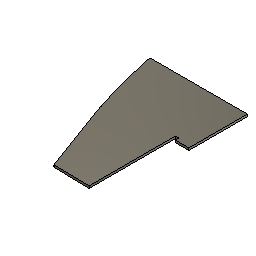
oceaan-25-floor_3 v6 (Autodesk Fusion 360 design; units mm, degrees)
Autodesk Fusion 360 part; units mm, degrees
note: some values were not read from the file. Set by a fixed rule: which sketch regions a step uses.
sketch "Sketch1" plane through (0, 0, 0) normal (0, 1, 0) x (1, 0, 0)
  line L0 (107.2779, 788.7865) -> (-437.7221, 788.7865)
  line L1 (12.2779, 481.7865) -> (31.2779, 481.7858)
  line L2 (31.2779, 481.7858) -> (31.1088, 461.7865)
  line L3 (31.1088, 461.7865) -> (107.2779, 461.7865)
  line L4 (12.2779, 481.7865) -> (12.2779, -0.2135)
  line L5 (-186.7221, 3.7865) -> (-186.7221, 419.7865)
  line L6 (-340.9767, 419.6292) -> (-188.1918, 3.7865)
  arc A0 (-437.7221, 788.7865) -> (-340.9767, 419.6292) centre (3793.4257, 1700.3924) ccw
  line L7 (12.2779, 788.7865) -> (107.2779, 788.7865)
  line L8 (12.2779, 788.7865) -> (107.2779, 788.7865)
  line L9 (107.2779, 788.7865) -> (107.2779, 481.7857)
  line L10 (107.2779, 481.7857) -> (107.2779, 461.7865)
  line L11 (12.2779, -0.2135) -> (-186.7221, 3.7865)
  line L12 (-186.7221, 3.7865) -> (-188.1918, 3.7865)
  dimension "d1" = 789
  dimension "d4" = 307
  dimension "d6" = 95
  dimension "d7" = 545
  dimension "d11" = 19
  dimension "d12" = 20
  dimension "d16" = 76
  constraint parallel L0 L8
  constraint perpendicular L3 L10
  measures "d1" distance of L4.end L7.start
  measures "d4" distance of L7.start L1.start
  measures "d6" distance of L7.start L0.start
  measures "d7" distance of L0.start L0.end
  measures "d11" distance of L1.start L1.end
  measures "d12" distance of L1.end L2.end
  measures "d16" distance of L1.end L9.end
extrude "Extrude1" add sketch "Sketch1" along normal blind 12.5
